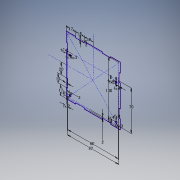
# Autodesk Inventor part: Back
Saved by Autodesk Inventor 2016 (Build 200138000, 138)
## iProperties
Created: 2017-05-22
Part Number: Back
Material: 一般
Document SubType Name: Modeling
Designer: KOTA-NPC2
Density: 1 g/cm^3
Appearance: 既定
Author: KOTA-NPC2
Autodesk Inventor part; units mm, degrees
ref_plane "YZ Plane" through (0, 0, 0) normal (1, 0, 0) x (0, 1, 0)
ref_plane "XZ Plane" through (0, 0, 0) normal (0, 1, 0) x (-1, 0, 0)
ref_plane "XY Plane" through (0, 0, 0) normal (0, 0, 1) x (1, 0, 0)
sketch "スケッチ1" plane through (0, 0, 0) normal (0, 1, 0) x (-1, 0, 0)
  line L0 (46, 50) -> (-46, 50) construction
  line L1 (-46, 50) -> (-46, -50) construction
  line L2 (-46, -50) -> (46, -50) construction
  line L3 (46, -50) -> (46, 50) construction
  line L4 (46, 50) -> (-46, -50) construction
  line L5 (-46, 50) -> (46, -50) construction
  circle A0 centre (41, -44) radius 1.5
  line L6 (45, 22) -> (-45, 22) construction
  line L7 (-45, 22) -> (-45, -48) construction
  line L8 (-45, -48) -> (45, -48) construction
  line L9 (45, -48) -> (45, 22) construction
  circle A1 centre (41, 18) radius 1.5
  circle A2 centre (-41, 18) radius 1.5
  circle A3 centre (-41, -44) radius 1.5
  line L10 (48, 0) -> (48, -20)
  line L11 (48, -20) -> (46, -20)
  line L12 (46, -20) -> (46, -35)
  line L13 (46, -35) -> (48, -35)
  line L14 (48, -35) -> (48, -52)
  line L15 (0, 0) -> (80.4536, 0) construction
  line L16 (48, 0) -> (48, 20)
  line L17 (48, 20) -> (46, 20)
  line L18 (46, 20) -> (46, 35)
  line L19 (46, 35) -> (48, 35)
  line L20 (48, 35) -> (48, 52)
  line L21 (0, 0) -> (0, 71.6244) construction
  line L22 (-48, 0) -> (-48, -20)
  line L23 (-48, -20) -> (-46, -20)
  line L24 (-46, -20) -> (-46, -35)
  line L25 (-46, -35) -> (-48, -35)
  line L26 (-48, -35) -> (-48, -52)
  line L27 (-48, 0) -> (-48, 20)
  line L28 (-48, 20) -> (-46, 20)
  line L29 (-46, 20) -> (-46, 35)
  line L30 (-46, 35) -> (-48, 35)
  line L31 (-48, 35) -> (-48, 52)
  line L32 (48, 52) -> (31, 52)
  line L33 (31, 52) -> (31, 50)
  line L34 (31, 50) -> (16, 50)
  line L35 (16, 50) -> (16, 52)
  line L36 (16, 52) -> (0, 52)
  line L37 (-48, 52) -> (-31, 52)
  line L38 (-31, 52) -> (-31, 50)
  line L39 (-31, 50) -> (-16, 50)
  line L40 (-16, 50) -> (-16, 52)
  line L41 (-16, 52) -> (0, 52)
  line L42 (46, -50) -> (-46, -50) construction
  line L43 (48, -52) -> (31, -52)
  line L44 (31, -52) -> (31, -50)
  line L45 (31, -50) -> (16, -50)
  line L46 (16, -50) -> (16, -52)
  line L47 (16, -52) -> (0, -52)
  line L48 (-16, -52) -> (0, -52)
  line L49 (-16, -50) -> (-16, -52)
  line L50 (-31, -50) -> (-16, -50)
  line L51 (-31, -52) -> (-31, -50)
  line L52 (-48, -52) -> (-31, -52)
  dimension "d0" = 92
  dimension "d1" = 100
  dimension "d2" = 3
  dimension "d5" = 90
  dimension "d6" = 70
  dimension "d7" = 1
  dimension "d8" = 2
  dimension "d9" = 3
  dimension "d10" = 4
  dimension "d11" = 4
  dimension "d12" = 4
  dimension "d13" = 4
  dimension "d14" = 3
  dimension "d15" = 3
  dimension "d16" = 4
  dimension "d17" = 4
  dimension "d18" = 4
  dimension "d19" = 4
  dimension "d32" = 17
  dimension "d33" = 15
  dimension "d34" = 20
  dimension "d35" = 2
  dimension "d36" = 2
  dimension "d37" = 17
  dimension "d38" = 15
  dimension "d39" = 16
  dimension "d40" = 2
  dimension "d41" = 2
  constraints: 106 end point, 29 symmetric about line, 9 perpendicular, 9 point on line, 4 centre point, 4 horizontal, 4 parallel, 2 midpoint, 1 vertical, 2 other
  measures "d0" distance of L2.end L1.end
  measures "d1" distance of L1.end L0.end
  measures "d2" diameter of A0
  measures "d5" distance of L8.end L7.end
  measures "d6" distance of L7.end L6.end
  measures "d7" distance between parallel lines of L1 L7
  measures "d8" distance between parallel lines of L2 L8
  measures "d9" diameter of A1
  measures "d10" distance from line of L9 A1.centre
  measures "d11" distance from line of L9 A0.centre
  measures "d12" distance from line of L8 A0.centre
  measures "d13" distance from line of L6 A1.centre
  measures "d14" diameter of A2
  measures "d15" diameter of A3
  measures "d16" distance from line of L7 A3.centre
  measures "d17" distance from line of L8 A3.centre
  measures "d18" distance from line of L7 A2.centre
  measures "d19" distance from line of L6 A2.centre
  measures "d32" distance of L13.end L14.end
  measures "d33" distance of L11.end L12.end
  measures "d34" distance of L10.start L10.end
  measures "d35" distance of L10.end L11.end
  measures "d36" distance between parallel lines of L3 L10
  measures "d37" distance of L20.end L32.end
  measures "d38" distance of L33.end L34.end
  measures "d39" distance of L35.end L36.end
  measures "d40" distance of L34.end L35.end
  measures "d41" distance between parallel lines of L0 L36
extrude "押し出し1" add sketch "スケッチ1" along normal mid plane 2
equation "\"d9\" = d2"
equation "\"d10\" = d11"
equation "\"d13\" = d12"
equation "\"d14\" = d2"
equation "\"d15\" = d2"
equation "\"d16\" = d11"
equation "\"d17\" = d10"
equation "\"d18\" = d11"
equation "\"d19\" = d10"
equation "\"d36\" = d35"
